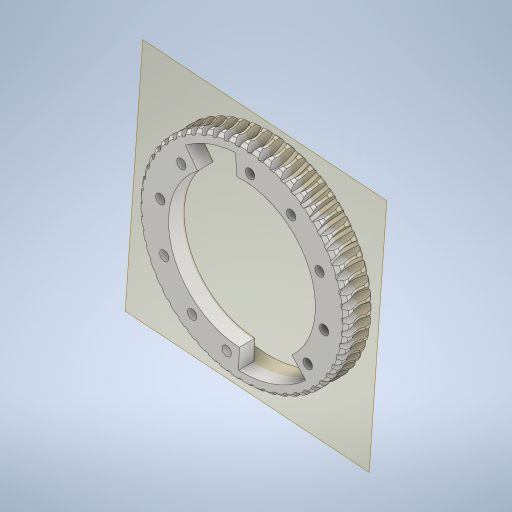
# Autodesk Inventor part: Worm Gear
Saved by Autodesk Inventor 2023.1 (Build 271208000, 208)
## iProperties
CustomPartVersion: 1
Created: 2022-12-25
Part Number: Worm Gear
Material: Steel, Mild
Document SubType Name: Modeling
Designer: USER
Categories: <?xml version="1.0" encoding="UTF-16"?> <MemberInstance><Categories><FamilyTemplate><FamilyTemplateParameter ValueType="xs:double" Id="1" ObjectReferenceKey="da_z" ObjectType="kUserParameterObject"/><FamilyTemplateParameter ValueType="xs:double" Id="2" ObjectReferenceKey="da_b" ObjectType="kUserParameterObject"/><FamilyTemplateParameter ValueType="xs:double" Id="3" ObjectReferenceKey="da_beta" ObjectType="kUserParameterObject"/><FamilyTemplateParameter ValueType="xs:double" Id="4" ObjectReferenceKey="da_m" ObjectType="kUserParameterObject"/><FamilyTemplateParameter ValueType="xs:double" Id="5" ObjectReferenceKey="da_alpha" ObjectType="kUserParameterObject"/><FamilyTemplateParameter ValueType="xs:double" Id="6" ObjectReferenceKey="da_da" ObjectType="kUserParameterObject"/><FamilyTemplateParameter ValueType="xs:double" Id="7" ObjectReferenceKey="da_aw" ObjectType="kUserParameterObject"/><FamilyTemplateParameter ValueType="xs:double" Id="8" ObjectReferenceKey="da_px" ObjectType="kUserParameterObject"/><FamilyTemplateParameter ValueType="xs:double" Id="9" ObjectReferenceKey="da_d" ObjectType="kUserParameterObject"/><FamilyTemplateParameter ValueType="xs:double" Id="10" ObjectReferenceKey="da_dae" ObjectType="kUserParameterObject"/><FamilyTemplateParameter ValueType="xs:double" Id="11" ObjectReferenceKey="da_fi" ObjectType="kUserParameterObject"/><FamilyTemplateParameter ValueType="xs:string" Id="12" ObjectReferenceKey="EAIAABAAAAAWFwAAAAAAAIAAAAAAAAAA" ObjectType="83910656" SubObjectId="SurfaceGeometry"/></FamilyTemplate><ParamToTemplateMap><ParamToTemplate CategoryParameter="//CategoryParameter[@InternalName='046C89C9-8512-4d59-83FE-43B91F4F132A']" TemplateParameter="1"/><ParamToTemplate CategoryParameter="//CategoryParameter[@InternalName='2552DF32-E462-4b46-AEBF-C6C7768E72AC']" TemplateParameter="2"/><ParamToTemplate CategoryParameter="//CategoryParameter[@InternalName='C9EE641D-15FC-4fae-A226-E94C4372FDD7']" TemplateParameter="3"/><ParamToTemplate><ParamToTemplate CategoryParameter="//CategoryParameter[@InternalName='00B6519A-459B-49c7-AD84-2E56D39A5744']" ConstantValue="0.173163"/></ParamToTemplate><ParamToTemplate><ParamToTemplate CategoryParameter="//CategoryParameter[@InternalName='04B31F0E-C7A6-4894-AA32-9629BEFACF47']" ConstantValue="1.000000"/></ParamToTemplate><ParamToTemplate><ParamToTemplate CategoryParameter="//CategoryParameter[@InternalName='43CBEC2E-7847-49e7-A936-2F7889FCB2D9']" ConstantValue="0.200000"/></ParamToTemplate><ParamToTemplate><ParamToTemplate CategoryParameter="//CategoryParameter[@InternalName='B1EFC894-105D-4ebd-86BF-FA20ED196853']" ConstantValue="0.300000"/></ParamToTemplate><ParamToTemplate><ParamToTemplate CategoryParameter="//CategoryParameter[@InternalName='51175063-3D10-4879-93E8-6246FE8B403D']" ConstantValue="2060000000.000000"/></ParamToTemplate><ParamToTemplate><ParamToTemplate CategoryParameter="//CategoryParameter[@InternalName='A3A52E27-4454-46a9-B0BD-C932399B70AF']" ConstantValue="0.300000"/></ParamToTemplate><ParamToTemplate CategoryParameter="//CategoryParameter[@InternalName='91B76062-C214-41d9-B1B9-14D2AB99603D']" TemplateParameter="4"/><ParamToTemplate CategoryParameter="//CategoryParameter[@InternalName='2D373A89-B862-43d6-8D0B-0CBF12AB9F6C']" TemplateParameter="5"/><ParamToTemplate CategoryParameter="//CategoryParameter[@InternalName='37777632-D6A2-4fac-9D53-DB8ACD95C989']" TemplateParameter="6"/><ParamToTemplate CategoryParameter="//CategoryParameter[@InternalName='FD1017F1-B727-4f7e-9707-0F86F1FF9423']" TemplateParameter="7"/><ParamToTemplate CategoryParameter="//CategoryParameter[@InternalName='3BF567DA-17EF-48d8-80EA-D119B07F6463']" TemplateParameter="8"/><ParamToTemplate CategoryParameter="//CategoryParameter[@InternalName='BF5A1E7E-5373-4a22-AAD3-F583781FCF3C']" TemplateParameter="9"/><ParamToTemplate CategoryParameter="//CategoryParameter[@InternalName='2A200944-5A8C-41ca-B96E-8520D2E510F1']" TemplateParameter="10"/><ParamToTemplate CategoryParameter="//CategoryParameter[@InternalName='E77AC4FD-7B43-4566-B0ED-7CA70B976BC8']" TemplateParameter="11"/><ParamToTemplate><ParamToTemplate CategoryParameter="//CategoryParameter[@InternalName='D4F72237-D604-435a-AD0B-F738B7463A00']" ConstantValue="110.000000"/></ParamToTemplate><ParamToTemplate><ParamToTemplate CategoryParameter="//CategoryParameter[@InternalName='9E1B4470-B2D3-4ff1-B813-535BB4CDF51A']" ConstantValue="2000000.000000"/></ParamToTemplate><ParamToTemplate><ParamToTemplate CategoryParameter="//CategoryParameter[@InternalName='A7A89E9A-52E6-4d4f-86CF-A81914F22AA4']" ConstantValue="250000000.000000"/></ParamToTemplate><ParamToTemplate><ParamToTemplate CategoryParameter="//CategoryParameter[@InternalName='B02FABAC-469F-4ad8-A219-DB4578299DF6']" ConstantValue="250000000.000000"/></ParamToTemplate><ParamToTemplate><ParamToTemplate CategoryParameter="//CategoryParameter[@InternalName='E6981962-40D5-4343-A0AD-C263FCC47E10']" ConstantValue="9.000000"/></ParamToTemplate><ParamToTemplate><ParamToTemplate CategoryParameter="//CategoryParameter[@InternalName='B958E99F-2BCD-4955-8634-793EB7B37B89']" ConstantValue="8.000000"/></ParamToTemplate><ParamToTemplate><ParamToTemplate CategoryParameter="//CategoryParameter[@InternalName='4AD49A87-569D-440f-A541-E3B52A6A9DCE']" ConstantValue="1200.000000"/></ParamToTemplate><ParamToTemplate><ParamToTemplate CategoryParameter="//CategoryParameter[@InternalName='4E5813A0-330D-4b41-BE23-D880B01A1D55']" ConstantValue="1650000.000000"/></ParamToTemplate><ParamToTemplate><ParamToTemplate CategoryParameter="//CategoryParameter[@InternalName='19EB8C86-AA88-4253-B4AA-2F5DF1CE171A']" ConstantValue="6000.000000"/></ParamToTemplate><ParamToTemplate CategoryParameter="//CategoryParameter[@InternalName='27C3BAF2-7550-4e4b-AE2C-0DB134B7D9B7']" TemplateParameter="12"/></ParamToTemplateMap><Category DisplayName="Gear" InternalName="DC85795E-93AB-48d5-8EEE-5A27447B64BD" Mnemonic="Gear"><CategoryParameter DisplayName="z" InternalName="046C89C9-8512-4d59-83FE-43B91F4F132A" Mnemonic="z"/><CategoryParameter DisplayName="b|.2|" InternalName="2552DF32-E462-4b46-AEBF-C6C7768E72AC" Mnemonic="b"/><CategoryParameter DisplayName="||b|" InternalName="C9EE641D-15FC-4fae-A226-E94C4372FDD7" Mnemonic="beta"/><CategoryParameter DisplayName="x" InternalName="00B6519A-459B-49c7-AD84-2E56D39A5744" Mnemonic="x"/><CategoryParameter DisplayName="a*" InternalName="04B31F0E-C7A6-4894-AA32-9629BEFACF47" Mnemonic="a"/><CategoryParameter DisplayName="c*" InternalName="43CBEC2E-7847-49e7-A936-2F7889FCB2D9" Mnemonic="c"/><CategoryParameter DisplayName="r|.f|*" InternalName="B1EFC894-105D-4ebd-86BF-FA20ED196853" Mnemonic="rf"/><CategoryParameter DisplayName="E" InternalName="51175063-3D10-4879-93E8-6246FE8B403D" Mnemonic="E"/><CategoryParameter DisplayName="||m|" InternalName="A3A52E27-4454-46a9-B0BD-C932399B70AF" Mnemonic="mi"/><Category DisplayName="WormGear" InternalName="1B25C7EF-093B-4025-B3D3-619CD2A4550C" Mnemonic="WormGear"><CategoryParameter DisplayName="m" InternalName="91B76062-C214-41d9-B1B9-14D2AB99603D" Mnemonic="m"/><CategoryParameter DisplayName="||a|" InternalName="2D373A89-B862-43d6-8D0B-0CBF12AB9F6C" Mnemonic="alpha"/><CategoryParameter DisplayName="d|.a|" InternalName="37777632-D6A2-4fac-9D53-DB8ACD95C989" Mnemonic="da"/><CategoryParameter DisplayName="a|.w|" InternalName="FD1017F1-B727-4f7e-9707-0F86F1FF9423" Mnemonic="aw"/><CategoryParameter DisplayName="p|.x|" InternalName="3BF567DA-17EF-48d8-80EA-D119B07F6463" Mnemonic="px"/><CategoryParameter DisplayName="d" InternalName="BF5A1E7E-5373-4a22-AAD3-F583781FCF3C" Mnemonic="d"/><CategoryParameter DisplayName="dae" InternalName="2A200944-5A8C-41ca-B96E-8520D2E510F1" Mnemonic="dae"/><CategoryParameter DisplayName="||d|" InternalName="E77AC4FD-7B43-4566-B0ED-7CA70B976BC8" Mnemonic="fi"/><CategoryParameter DisplayName="VHV" InternalName="D4F72237-D604-435a-AD0B-F738B7463A00" Mnemonic="VHV"/><CategoryParameter DisplayName="||s||.Hlim|" InternalName="9E1B4470-B2D3-4ff1-B813-535BB4CDF51A" Mnemonic="sHlim"/><CategoryParameter DisplayName="N|.Flim|" InternalName="A7A89E9A-52E6-4d4f-86CF-A81914F22AA4" Mnemonic="NFlim"/><CategoryParameter DisplayName="N|.Hlim|" InternalName="B02FABAC-469F-4ad8-A219-DB4578299DF6" Mnemonic="NHlim"/><CategoryParameter DisplayName="q|.F|" InternalName="E6981962-40D5-4343-A0AD-C263FCC47E10" Mnemonic="qF"/><CategoryParameter DisplayName="q|.H|" InternalName="B958E99F-2BCD-4955-8634-793EB7B37B89" Mnemonic="qH"/><CategoryParameter DisplayName="v|.max|" InternalName="4AD49A87-569D-440f-A541-E3B52A6A9DCE" Mnemonic="maxv"/><CategoryParameter DisplayName="S|.n|" InternalName="4E5813A0-330D-4b41-BE23-D880B01A1D55" Mnemonic="Sn"/><CategoryParameter DisplayName="K|.w|" InternalName="19EB8C86-AA88-4253-B4AA-2F5DF1CE171A" Mnemonic="Kw"/><CategoryParameter DisplayName="PitchDiameter" InternalName="27C3BAF2-7550-4e4b-AE2C-0DB134B7D9B7" Mnemonic="IDS_PITCHDIAM"/></Category></Category></Categories></MemberInstance>
Density: 7.86 g/cm^3
Appearance: Steel
Author: USER
## iProperties of the stored document Worm Gear2_3DPrint.ipt
Created: 2022-12-25
Part Number: Worm Gear2_3DPrint
Material: Generic
Document SubType Name: Modeling
Designer: USER
Density: 1 g/cm^3
Appearance: Default
Author: USER
Autodesk Inventor part; units mm, degrees
ref_plane "Tooth Plane" through (0, -10, 0) normal (-0.1104315, 0, 0.9938837) x (0, 1, 0)
sketch "Base Body Sketch" plane through (0, 0, 0) normal (1, 0, 0) x (0, 1, 0)
  line L0 (0, -8.82) -> (0, 8.82) projected
  line L1 (0, 6.3) -> (45.333, 6.3)
  line L2 (45.333, 6.3) -> (46.6771, 4.9218)
  line L3 (-11.4154, 0) -> (68.4925, 0) construction
  circle A0 centre (51.4771, 0) radius 5.6
  line L4 (46.6771, 4.9218) -> (46.6771, -4.9218)
  line L5 (0, -6.3) -> (45.333, -6.3)
  line L6 (0, 6.3) -> (0, -6.3)
  line L7 (45.333, -6.3) -> (46.6771, -4.9218)
  dimension "d50" = 45.718
  dimension "d87" = 93.3541
  dimension "d89" = 11.2
  dimension "d92" = 12.6
  dimension "d93" = 51.4771
  constraints: 14 end point, 3 symmetric about line, 2 perpendicular, 2 point on line, 1 centre point, 1 collinear
  measures "d50" angle of L2 L1
  measures "d87" diameter of L4 L0
  measures "d89" diameter of A0
  measures "d92" distance of L1.start L5.start
  measures "d93" distance from line of A0.centre L6
revolve "Base Body" add sketch "Base Body Sketch" angle 360 about axis through (0, 0, 0) along (0, 0, 1) picked at (46.5079, -0.5954) contours L0 L1 L2 L4 A0 L7 L5 | A0 L4
revolve "Base Body2" cut sketch "Base Body Sketch" angle 360 about axis through (0, 0, 0) along (0, 0, 1) contours L4 A0 | A0 L4
sketch "Tooth Sketch" plane through (0, -10, 0) normal (-0.1104315, 0, 0.9938837) x (0, 1, 0)
  line L0 (10, 3.0895) -> (10, -3.0895) projected
  line L1 (-43.3011, 0) -> (-30.5331, 0) projected
  line L2 (-41.4771, 2.2068) -> (-41.4771, -2.2068)
  line L3 (-41.4771, -2.2068) -> (-36.1971, -2.2068)
  line L4 (-36.1971, -2.2068) -> (-32.3571, -0.8091)
  line L5 (-32.3571, -0.8091) -> (-32.3571, 0)
  line L6 (-32.3571, 0.8091) -> (-36.1971, 2.2068)
  line L7 (-36.1971, 2.2068) -> (-41.4771, 2.2068)
  line L8 (-32.3571, 0.8091) -> (-32.3571, 0)
  line L9 (-34.2771, 0) -> (-34.2771, -1.508) construction
  dimension "d38" = 51.4771
  dimension "d39" = 20
  dimension "d40" = 5.28
  dimension "d41" = 7.2
  dimension "d42" = 1.508
  constraints: 16 end point, 4 perpendicular, 3 equal length, 2 point on line, 1 midpoint, 1 parallel, 1 vertical
  measures "d38" distance between parallel lines of L0 L2
  measures "d39" angle of L6 L7
  measures "d40" distance of L6.end L2.start
  measures "d41" distance between parallel lines of L2 L9
  measures "d42" distance of L9.start L9.end
sketch "Sketch8" plane through (0, 0, 6.3) normal (0, 0, 1) x (1, 0, 0)
  circle A0 centre (0, 0) radius 45.333 projected
  circle A1 centre (0, 0) radius 44
  dimension "d77" = 88
  constraints: 1 centre point, 1 coincident
  measures "d77" diameter of A1
surface extrude "Pitch Diameter" sketch "Sketch8" against normal blind 12.6 shown no curves A1
ref_plane "Work Plane13" through (0, 0, 0) normal (-0.0570888, 0.9983691, 0) x (0, 0, 1)
revolve "Tooth" cut sketch "Tooth Sketch" angle 360 about axis through (-2.1933, -51.4771, -0.2437) along (0.9938837, 0, 0.1104315)
pattern_circular "Tooth Pattern" count 55 over 360 about axis through (0, 0, 0) along (0, 0, 1) of "Tooth"
ref_plane "Work Plane14" through (0, 0, 0) normal (0.9983691, 0.0570888, 0) x (0, 0, 1)
ref_plane "Work Plane15" through (0, 0, 0) normal (0, -1, 0) x (0, 0, 1)
sketch "Sketch9" plane through (0, 0, -6.3) normal (0, 0, -1) x (-0.9877666, 0.1559395, 0)
  circle A0 centre (0, 0) radius 42.0487
  ellipse E0 centre (-51.2908, 4.4488) end of major axis (-42.1937, 3.8027) minor radius 1.0071 (-44.7136, 3.2899) -> (-44.7878, 4.6987) ccw
  constraints: 1 centre point, 1 coincident, 4 other
extrude "Extrusion1" cut sketch "Sketch9" against normal blind 21.25
ref_plane "Work Plane16" through (0, 0, 0) normal (0, 0, 1) x (0.9974162, -0.071839, 0)
sketch "Sketch11" plane through (0, 0, 6.3) normal (0, 0, 1) x (0.9974162, -0.071839, 0)
  circle A0 centre (0, 0) radius 42.0487 projected
  line L0 (0, 0) -> (1.5109, -42.0215)
  line L1 (0, 0) -> (30.7317, -28.6994)
  line L2 (0, 0) -> (-27.6955, 31.6394)
  line L3 (0, 0) -> (-5.9142, 41.6307)
  circle A1 centre (0, 0) radius 32.9825
  point P0 (1.1851, -32.9612)
  point P1 (-21.7241, 24.8176)
  point P2 (-4.6391, 32.6547)
  point P3 (24.1056, -22.5115)
  constraints: 8 end point, 4 point on circle, 1 centre point, 1 coincident
extrude "Extrusion3" add sketch "Sketch11" against normal blind 7 contours A0 L1 A1 L3 | L2 A1 L0 A0
sketch "Sketch12" plane through (0, 0, -0.7) normal (0, 0, -1) x (-0.9974162, 0.071839, 0)
  point P0 (0, 0)
  point P1 (33.7416, -16.5907)
hole "Hole3" at (-34.8463, -14.1239, -0.7) direction (0, 0, 1) diameter 4.2 depth 8
sketch "Sketch13" plane through (0, 0, -0.7) normal (0, 0, -1) x (-0.9974162, 0.071839, 0)
  point P0 (0, 0)
  point P1 (-33.7149, 17.0942)
  point P2 (-1.0168, 37.1772)
  point P3 (-31.2131, -21.7865)
  point P4 (-37.2949, -4.4401)
  point P5 (-19.8669, 31.6836)
  point P6 (28.9316, 23.3995)
  point P7 (4.133, -37.5411)
  point P8 (20.0458, -32.2285)
  point P9 (37.0359, 4.3814)
hole "Hole4" at (34.8558, 14.628, -0.7) at (3.685, 37.0081, -0.7) at (29.5674, -23.9725, -0.7) at (36.8796, -7.1078, -0.7) at (22.0916, 30.1745, -0.7) at (-27.1758, 25.4174, -0.7) at (-6.8192, -37.1472, -0.7) at (-22.3093, -30.7052, -0.7) at (-36.6254, 7.0307, -0.7) direction (0, 0, 1) diameter 4.2 depth 8
equation "\"d50\" = da_fi"
equation "\"d87\" = da_dae"
equation "\"d89\" = 2 * da_aw - da_da"
equation "\"d92\" = da_b"
equation "\"d93\" = da_aw"
equation "\"d38\" = da_aw"
equation "\"d39\" = da_alfat"
equation "\"d40\" = 0.5 * da_df1"
equation "\"d41\" = 0.5 * da_d1"
equation "\"d42\" = 0.3 * da_px"
equation "\"d77\" = da_dw"
equation "\"d78\" = da_b"
equation "\"da_aw\" = 51.47706"
equation "\"da_fi\" = 45.7178deg"
equation "\"da_b\" = 12.6"
equation "\"da_df\" = 84.71412"
equation "\"da_da\" = 91.75412"
equation "\"da_beta\" = 6.340192deg"
equation "\"da_alfat\" = 20deg"
equation "\"da_df1\" = 10.56"
equation "\"da_da1\" = 17.6"
equation "\"da_d1\" = 14.4"
equation "\"da_px\" = 5.02655"
equation "\"d68\" = da_aw"
equation "\"da_dw\" = 88"
equation "\"da_rightdir\" = 0"
equation "\"d86\" = da_aw"
equation "\"da_dae\" = 93.35412"
body "Solid1"
body "Srf1"
